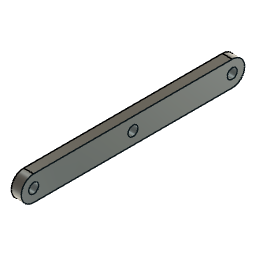
brazos v3 elevador camara (Autodesk Fusion 360 design; units mm, degrees)
Autodesk Fusion 360 part; units mm, degrees
sketch "Sketch1" plane through (0, 0, 0) normal (1, 0, 0) x (0, 1, 0)
  circle A0 centre (0, 0) radius 5
  line L0 (0, 5) -> (80, 5)
  line L1 (0, -5) -> (80, -5)
  circle A1 centre (80, 0) radius 5
  dimension "d1" = 10
  dimension "d2" = 80
  constraint coincident A0.centre origin
  constraint coincident A0 L0.start
  constraint horizontal L0
  constraint coincident A0 L1.start
  constraint tangent A0 L1
  constraint parallel L0 L1
  constraint coincident L0.end A1
  constraint tangent L0 A1
  measures "d1" diameter of A0
  measures "d2" distance of L0.start L0.end
extrude "Extrude1" add sketch "Sketch1" along normal blind 4
sketch "Sketch2" plane through (4, 0, 0) normal (1, 0, 0) x (0, 1, 0)
  arc A0 (0, 5) -> (0, -5) centre (0, 0) ccw
  line L0 (0, -5) -> (80, -5)
  arc A1 (80, -5) -> (80, 5) centre (80, 0) ccw
  line L1 (80, 5) -> (0, 5)
  circle A2 centre (0, 0) radius 2
  circle A3 centre (80, 0) radius 2
  dimension "d5" = 4
  dimension "d6" = 4
  constraint coincident A0.centre A2.centre
  constraint concentric A1 A3
  measures "d5" diameter of A2
  measures "d6" diameter of A3
extrude "Extrude2" cut sketch "Sketch2" against normal blind 20 contours A2 | A3
sketch "Sketch3" plane through (4, 0, 0) normal (1, 0, 0) x (0, 1, 0)
  circle A0 centre (0, 0) radius 2
  circle A1 centre (80, 0) radius 2
  arc A2 (0, 5) -> (0, -5) centre (0, 0) ccw
  line L0 (0, -5) -> (80, -5)
  arc A3 (80, -5) -> (80, 5) centre (80, 0) ccw
  line L1 (80, 5) -> (0, 5)
  circle A4 centre (40, 0) radius 2
  dimension "d9" = 4
  measures "d9" diameter of A4
extrude "Extrude3" cut sketch "Sketch3" against normal blind 20 contours A4
sketch "Sketch4" plane through (0, 0, 0) normal (0, 0, 1) x (1, 0, 0)
sketch "Sketch5" plane through (4, 0, 0) normal (1, 0, 0) x (0, 1, 0)
  circle A0 centre (40, 0) radius 2
  circle A1 centre (0, 0) radius 2
  circle A2 centre (80, 0) radius 2
  arc A3 (0, 5) -> (0, -5) centre (0, 0) ccw
  line L0 (0, -5) -> (80, -5)
  arc A4 (80, -5) -> (80, 5) centre (80, 0) ccw
  line L1 (80, 5) -> (0, 5)
